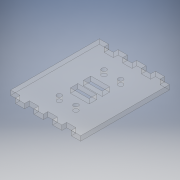
# Autodesk Inventor part: top
Saved by Autodesk Inventor 2018 (Build 220112000, 112)
## iProperties
Created: 2018-12-08
Part Number: top
Material: Polycarbonate, Clear
Document SubType Name: Modeling
Designer: Jayden
Density: 1.2 g/cm^3
Appearance: Polycarbonate - Clear
Author: Jayden
Autodesk Inventor part; units mm, degrees
ref_plane "YZ Plane" through (0, 0, 0) normal (1, 0, 0) x (0, 1, 0)
ref_plane "XZ Plane" through (0, 0, 0) normal (0, 1, 0) x (-1, 0, 0)
ref_plane "XY Plane" through (0, 0, 0) normal (0, 0, 1) x (1, 0, 0)
sketch "Sketch1" plane through (0, 0, 0) normal (0, 1, 0) x (-1, 0, 0)
  line L0 (38.1, 13.317) -> (50.8, 13.317)
  line L1 (25.4, 13.317) -> (25.4, 19.667)
  line L2 (25.4, 19.667) -> (38.1, 19.667)
  line L3 (38.1, 19.667) -> (38.1, 13.317)
  line L4 (12.7, 19.667) -> (12.7, 13.317)
  line L5 (12.7, 13.317) -> (25.4, 13.317)
  line L6 (25.4, 13.317) -> (25.4, 19.667)
  line L7 (12.7, 19.667) -> (0, 19.667)
  line L8 (0, 19.667) -> (0, 13.317)
  line L9 (12.7, 13.317) -> (12.7, 19.667)
  line L10 (-12.7, 19.667) -> (-12.7, 13.317)
  line L11 (-12.7, 13.317) -> (0, 13.317)
  line L12 (0, 13.317) -> (0, 19.667)
  line L13 (-12.7, 19.667) -> (-25.4, 19.667)
  line L14 (-25.4, 19.667) -> (-25.4, 13.317)
  line L15 (-12.7, 13.317) -> (-12.7, 19.667)
  line L16 (-38.1, 19.667) -> (-38.1, 13.317)
  line L17 (-38.1, 13.317) -> (-25.4, 13.317)
  line L18 (-25.4, 13.317) -> (-25.4, 19.667)
  line L19 (-38.1, 19.667) -> (-50.8, 19.667)
  line L20 (-50.8, 19.667) -> (-50.8, 13.317)
  line L21 (-38.1, 13.317) -> (-38.1, 19.667)
  line L22 (38.1, -107.333) -> (50.8, -107.333)
  line L23 (38.1, -100.983) -> (25.4, -100.983)
  line L24 (12.7, -107.333) -> (25.4, -107.333)
  line L25 (-12.7, -100.983) -> (-25.4, -100.983)
  line L26 (-25.4, -107.333) -> (-38.1, -107.333)
  line L27 (-38.1, -107.333) -> (-38.1, -100.983)
  line L28 (-38.1, -100.983) -> (-50.8, -100.983)
  line L29 (-25.4, -100.983) -> (-25.4, -107.333)
  line L30 (12.7, -100.983) -> (0, -100.983)
  line L31 (-12.7, -107.333) -> (-12.7, -100.983)
  line L32 (-12.7, -107.333) -> (0, -107.333)
  line L33 (0, -100.983) -> (0, -107.333)
  line L34 (12.7, -107.333) -> (12.7, -100.983)
  line L35 (25.4, -100.983) -> (25.4, -107.333)
  line L36 (38.1, -107.333) -> (38.1, -100.983)
  line L37 (-50.8, 13.317) -> (-38.1, 13.317) construction
  line L38 (50.8, -107.333) -> (50.8, 13.317)
  line L39 (-50.8, 13.317) -> (-50.8, -100.983)
  line L40 (12.7, -40.023) -> (-12.7, -40.023)
  line L41 (-12.7, -40.023) -> (-12.7, -29.863)
  line L42 (-12.7, -29.863) -> (12.7, -29.863)
  line L43 (12.7, -29.863) -> (12.7, -40.023)
  line L44 (12.7, -57.803) -> (-12.7, -57.803)
  line L45 (-12.7, -57.803) -> (-12.7, -47.643)
  line L46 (-12.7, -47.643) -> (12.7, -47.643)
  line L47 (12.7, -47.643) -> (12.7, -57.803)
  line L48 (0, 13.317) -> (0, -29.863) construction
  circle A0 centre (11.35, -74.303) radius 3.175
  circle A1 centre (-11.35, -74.303) radius 3.175
  circle A2 centre (11.35, -13.363) radius 3.175
  circle A3 centre (-11.35, -13.363) radius 3.175
  point P0 (0, 0)
  dimension "d4" = 12.7
  dimension "d6" = 12.7
  dimension "d7" = 6.35
  dimension "d8" = 12.7
  dimension "d9" = 6.35
  dimension "d10" = 12.7
  dimension "d11" = 6.35
  dimension "d12" = 12.7
  dimension "d13" = 6.35
  dimension "d14" = 12.7
  dimension "d15" = 6.35
  dimension "d16" = 12.7
  dimension "d17" = 6.35
  dimension "d21" = 12.7
  dimension "d22" = 12.7
  dimension "d23" = 12.7
  dimension "d24" = 12.7
  dimension "d25" = 12.7
  dimension "d27" = 12.7
  dimension "d28" = 12.7
  dimension "d31" = 6.35
  dimension "d35" = 12.7
  dimension "d39" = 6.35
  dimension "d40" = 6.35
  dimension "d43" = 6.35
  dimension "d45" = 6.35
  dimension "d46" = 12.7
  dimension "d47" = 6.35
  dimension "d53" = 90
  dimension "d54" = 90
  dimension "d55" = 90
  dimension "d56" = 90
  dimension "d57" = 90
  dimension "d58" = 90
  dimension "d59" = 90
  dimension "d60" = 90
  dimension "d61" = 90
  dimension "d62" = 90
  dimension "d63" = 90
  dimension "d64" = 90
  dimension "d65" = 90
  dimension "d68" = 6.35
  dimension "d69" = 6.35
  dimension "d70" = 6.35
  dimension "d71" = 0
  dimension "d72" = 90
  dimension "d73" = 90
  dimension "d74" = 90
  dimension "d75" = 90
  dimension "d76" = 90
  dimension "d77" = 90
  dimension "d78" = 90
  dimension "d79" = 90
  dimension "d80" = 90
  dimension "d81" = 90
  dimension "d82" = 90
  dimension "d83" = 90
  dimension "d84" = 90
  dimension "d86" = 127
  dimension "d89" = 25.4
  dimension "d90" = 10.16
  dimension "d92" = 38.1
  dimension "d93" = 25.4
  dimension "d94" = 10.16
  constraints: 98 end point, 11 parallel, 6 horizontal, 5 perpendicular, 4 centre point, 1 midpoint, 1 point on line, 1 vertical
  measures "d4" distance of L0.end L0.start
  measures "d6" distance of L1.end L2.end
  measures "d7" distance of L1.start L1.end
  measures "d8" distance of L5.end L4.end
  measures "d9" distance of L4.end L4.start
  measures "d10" distance of L8.end L9.start
  measures "d11" distance of L8.end L7.end
  measures "d12" distance of L10.end L8.end
  measures "d13" distance of L10.end L10.start
  measures "d14" distance of L10.end L14.end
  measures "d15" distance of L14.end L13.end
  measures "d16" distance of L17.end L16.end
  measures "d17" distance of L16.end L16.start
  measures "d21" distance of L30.start L33.start
  measures "d22" distance of L23.start L35.start
  measures "d23" distance of L22.start L22.end
  measures "d24" distance of L24.start L24.end
  measures "d25" distance of L31.start L33.end
  measures "d27" distance of L27.end L28.end
  measures "d28" distance of L31.end L29.start
  measures "d31" distance between parallel lines of L28 L26
  measures "d35" distance of L16.start L19.end
  measures "d39" distance of L22.start L23.start
  measures "d40" distance of L35.start L24.end
  measures "d43" distance of L31.start L31.end
  measures "d45" distance of L27.start L27.end
  measures "d46" distance of L29.end L27.start
  measures "d47" distance of L2.end L0.start
  measures "d53" angle of L3 L0
  measures "d54" angle of L2 L3
  measures "d55" angle of L2 L6
  measures "d56" angle of L1 L5
  measures "d57" angle of L4 L5
  measures "d58" angle of L7 L4
  measures "d59" angle of L7 L8
  measures "d60" angle of L8 L11
  measures "d61" angle of L15 L13
  measures "d62" angle of L13 L18
  measures "d63" angle of L14 L17
  measures "d64" angle of L17 L16
  measures "d65" angle of L19 L21
  measures "d68" distance of L29.start L29.end
  measures "d69" distance of L33.start L33.end
  measures "d70" distance of L24.start L30.start
  measures "d71" horizontal distance of L0.end L22.end
  measures "d72" angle of L36 L22
  measures "d73" angle of L36 L23
  measures "d74" angle of L35 L23
  measures "d75" angle of L35 L24
  measures "d76" angle of L24 L34
  measures "d77" angle of L34 L30
  measures "d78" angle of L30 L33
  measures "d79" angle of L33 L32
  measures "d80" angle of L32 L31
  measures "d81" angle of L25 L31
  measures "d82" angle of L25 L29
  measures "d83" angle of L29 L26
  measures "d84" angle of L26 L27
  measures "d86" distance from line of L2 L22.end
  measures "d89" distance of L41.end L42.end
  measures "d90" distance of L40.end L41.end
  measures "d92" distance between parallel lines of L39 L41
  measures "d93" distance of L45.end L46.end
  measures "d94" distance of L44.end L45.end
extrude "Extrusion3" add sketch "Sketch1" along normal blind 6.35
body "Solid3"
